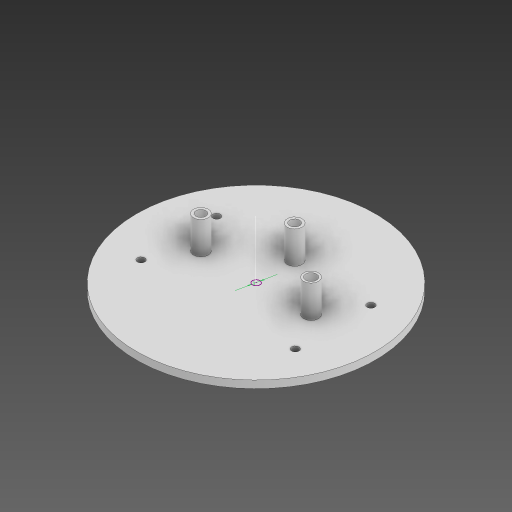
# Autodesk Inventor part: openmv
Saved by Autodesk Inventor 2023 (Build 270158000, 158)
## iProperties
Created: 2025-06-30
Part Number: openmv
Material: Типовые
Document SubType Name: Modeling
Designer: daa
Density: 1 g/cm^3
Appearance: По умолчанию
Author: daa
Autodesk Inventor part; units mm, degrees
ref_plane "YZ Plane" through (0, 0, 0) normal (1, 0, 0) x (0, 1, 0)
ref_plane "XZ Plane" through (0, 0, 0) normal (0, 1, 0) x (-1, 0, 0)
ref_plane "XY Plane" through (0, 0, 0) normal (0, 0, 1) x (1, 0, 0)
sketch "Эскиз1" plane through (0, 0, 0) normal (0, 1, 0) x (-1, 0, 0)
  circle A0 centre (0, 0) radius 48
  line L0 (31, 15.207) -> (-31, 15.207)
  line L1 (-31, 15.207) -> (-31, -15.207)
  line L2 (-31, -15.207) -> (31, -15.207)
  line L3 (31, -15.207) -> (31, 15.207)
  circle A1 centre (31, 15.207) radius 1.5
  circle A2 centre (31, -15.207) radius 1.5
  circle A3 centre (-31, 15.207) radius 1.5
  circle A4 centre (-31, -15.207) radius 1.5
  dimension "d0" = 96
  dimension "d1" = 62
  dimension "d2" = 30.414
  dimension "d3" = 31
  dimension "d4" = 15.207
  dimension "d5" = 3
  dimension "d6" = 3
  dimension "d7" = 3
  dimension "d8" = 3
  constraints: 8 end point, 5 centre point, 5 coincident, 2 parallel, 1 horizontal, 1 perpendicular
  measures "d0" diameter of A0
  measures "d1" distance of L2.end L1.end
  measures "d2" distance of L1.end L0.end
  measures "d3" horizontal distance of L2.end point (0, 0)
  measures "d4" vertical distance of point (0, 0) L0.end
  measures "d5" diameter of A1
  measures "d6" diameter of A2
  measures "d7" diameter of A3
  measures "d8" diameter of A4
extrude "Выдавливание1" add sketch "Эскиз1" along normal blind 3 contours A0 | L0 A1 L3 A2 L2 A4 L1 A3
sketch "Эскиз2" plane through (0, 3, 0) normal (0, 1, 0) x (1, 0, 0)
  circle A0 centre (0, 0) radius 27.25
  circle A1 centre (-22.15, 0) radius 3
  circle A2 centre (22.15, 0) radius 3
  circle A3 centre (0, 15.543) radius 3
  dimension "d11" = 54.5
  dimension "d12" = 6
  dimension "d13" = 6
  dimension "d14" = 44.3
  dimension "d15" = 22.15
  dimension "d16" = 6
  dimension "d17" = 15.543
  constraints: 4 centre point, 1 coincident
  measures "d11" diameter of A0
  measures "d12" diameter of A1
  measures "d13" diameter of A2
  measures "d14" distance of A2.centre A1.centre
  measures "d15" distance of point (0, 0) A1.centre
  measures "d16" diameter of A3
  measures "d17" distance of point (0, 0) A3.centre
extrude "Выдавливание2" add sketch "Эскиз2" along normal blind 13 contours A1 | A2 | A3
sketch "Эскиз3" plane through (0, 16, -15.543) normal (0, 1, 0) x (-1, 0, 0)
  circle A0 centre (0, 0) radius 2
  circle A1 centre (-22.15, 15.543) radius 2.2
  circle A2 centre (22.15, 15.543) radius 2
  circle A3 centre (22.15, 15.543) radius 3
  circle A4 centre (22.15, 15.543) radius 3 projected
  circle A5 centre (0, 0) radius 3
  circle A6 centre (0, 0) radius 3 projected
  circle A7 centre (-22.15, 15.543) radius 3
  circle A8 centre (-22.15, 15.543) radius 3 projected
  point P0 (0, 15.543)
  dimension "d20" = 4
  dimension "d21" = 4.4
  dimension "d22" = 4
  dimension "d23" = 6
  dimension "d24" = 6
  dimension "d25" = 6
  constraints: 6 centre point, 3 coincident, 3 concentric
  measures "d20" diameter of A0
  measures "d21" diameter of A1
  measures "d22" diameter of A2
  measures "d23" diameter of A3
  measures "d24" diameter of A5
  measures "d25" diameter of A7
extrude "Выдавливание3" cut sketch "Эскиз3" against normal blind 5 contours A0 | A1 | A2
sketch "Эскиз4" plane through (0, 3, 0) normal (0, 1, 0) x (1, 0, 0)
  circle A0 centre (0, 0) radius 1.5
  dimension "d28" = 3
  constraints: 1 centre point, 1 coincident
  measures "d28" diameter of A0
